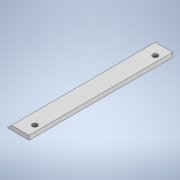
# Autodesk Inventor part: Cuchilla Versión 1
Saved by Autodesk Inventor 2020 (Build 240168000, 168)
## iProperties
Created: 2021-08-16
Part Number: Cuchilla Versión 1
Material: Generic
Document SubType Name: Modeling
Designer: Judac
Density: 1 g/cm^3
Appearance: Default
Author: Judac
Autodesk Inventor part; units mm, degrees
ref_plane "YZ Plane" through (0, 0, 0) normal (1, 0, 0) x (0, 1, 0)
ref_plane "XZ Plane" through (0, 0, 0) normal (0, 1, 0) x (-1, 0, 0)
ref_plane "XY Plane" through (0, 0, 0) normal (0, 0, 1) x (1, 0, 0)
sketch "Sketch1" plane through (0, 0, 0) normal (0, 1, 0) x (-1, 0, 0)
  line L0 (0, 0) -> (15, 0)
  line L1 (15, 0) -> (15, -99)
  line L2 (15, -99) -> (0, -99)
  line L3 (0, -99) -> (0, 0)
  circle A0 centre (4, -8) radius 1.75
  circle A1 centre (4, -91) radius 1.75
  dimension "d0" = 99
  dimension "d1" = 15
  dimension "d2" = 8
  dimension "d3" = 83
  dimension "d4" = 4
  dimension "d5" = 4
  dimension "d6" = 3.5
  dimension "d7" = 3.5
  constraints: 8 end point, 2 centre point, 2 parallel, 1 horizontal, 1 perpendicular
  measures "d0" distance of L0.end L1.end
  measures "d1" distance of L0.start L0.end
  measures "d2" distance from line of L0 A0.centre
  measures "d3" distance of A1.centre A0.centre
  measures "d4" distance from line of L3 A0.centre
  measures "d5" distance from line of L3 A1.centre
  measures "d6" diameter of A0
  measures "d7" diameter of A1
extrude "Extrusion1" add sketch "Sketch1" along normal blind 3
sketch "Sketch2" plane through (-15, 0, 0) normal (0, 0, 1) x (1, 0, 0)
  line L0 (0, 0) -> (3, 3)
  line L1 (0, 0) -> (15, 0) projected
  line L2 (0, 3) -> (15, 3) projected
  line L3 (3, 3) -> (0, 3)
  line L4 (0, 3) -> (0, 0)
  dimension "d10" = 45
  constraints: 6 end point, 1 horizontal, 1 perpendicular, 1 point on line
  measures "d10" angle of L1 L0
extrude "Extrusion2" cut sketch "Sketch2" against normal up to surface (99 mm away)
body "Solid1"
